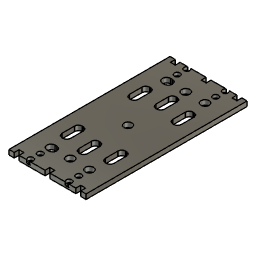
FS80+UL Pivot Base v20 (Autodesk Fusion 360 design; units mm, degrees)
Autodesk Fusion 360 part; units mm, degrees
note: some values were not read from the file. Set by a fixed rule: which sketch regions a step uses.
sketch "Schizzo5" plane through (0, 0, 0) normal (0, 0, 1) x (1, 0, 0)
  line L0 (214.6877, 113.6857) -> (294.6877, 113.6857)
  line L1 (294.6877, 113.6857) -> (294.6877, -53.5143)
  line L2 (294.6877, -53.5143) -> (214.6877, -53.5143)
  line L3 (214.6877, -53.5143) -> (214.6877, 113.6857)
  line L4 (254.6877, 113.6857) -> (254.6877, -53.5143) construction
  line L5 (214.6877, 30.0857) -> (294.6877, 30.0857) construction
  line L6 (274.6877, -51.0143) -> (234.6877, -51.0143) construction
  line L7 (234.6877, -51.0143) -> (234.6877, -41.0143) construction
  line L8 (234.6877, -41.0143) -> (274.6877, -41.0143) construction
  line L9 (274.6877, -41.0143) -> (274.6877, -51.0143) construction
  line L10 (274.6877, -51.0143) -> (234.6877, -41.0143) construction
  line L11 (234.6877, -51.0143) -> (274.6877, -41.0143) construction
  line L12 (225.2377, -53.5143) -> (220.1377, -53.5143)
  line L13 (220.1377, -53.5143) -> (220.1377, -48.5143)
  line L14 (220.1377, -48.5143) -> (225.2377, -48.5143)
  line L15 (225.2377, -48.5143) -> (225.2377, -53.5143)
  line L16 (225.2377, -53.5143) -> (220.1377, -48.5143) construction
  line L17 (220.1377, -53.5143) -> (225.2377, -48.5143) construction
  line L18 (289.2377, -48.5143) -> (284.1377, -48.5143)
  line L19 (289.2377, -53.5143) -> (289.2377, -48.5143)
  line L20 (284.1377, -48.5143) -> (284.1377, -53.5143)
  line L21 (284.1377, -53.5143) -> (289.2377, -53.5143)
  circle A0 centre (234.6877, -41.0143) radius 1.6
  circle A1 centre (234.6877, -41.0143) radius 2.95
  line L22 (234.6877, -46.0143) -> (274.6877, -46.0143) construction
  circle A2 centre (234.6877, -51.0143) radius 1.6
  circle A3 centre (234.6877, -51.0143) radius 2.95
  circle A4 centre (274.6877, -41.0143) radius 2.95
  circle A5 centre (274.6877, -41.0143) radius 1.6
  circle A6 centre (274.6877, -51.0143) radius 1.6
  circle A7 centre (274.6877, -51.0143) radius 2.95
  circle A8 centre (234.6877, 111.1857) radius 2.95
  circle A9 centre (234.6877, 111.1857) radius 1.6
  circle A10 centre (234.6877, 101.1857) radius 2.95
  circle A11 centre (234.6877, 101.1857) radius 1.6
  circle A12 centre (274.6877, 101.1857) radius 2.95
  circle A13 centre (274.6877, 101.1857) radius 1.6
  circle A14 centre (274.6877, 111.1857) radius 2.95
  circle A15 centre (274.6877, 111.1857) radius 1.6
  line L23 (289.2377, 108.6857) -> (284.1377, 108.6857)
  line L24 (284.1377, 108.6857) -> (284.1377, 113.6857)
  line L25 (289.2377, 113.6857) -> (289.2377, 108.6857)
  line L26 (225.2377, 108.6857) -> (225.2377, 113.6857)
  line L27 (220.1377, 108.6857) -> (225.2377, 108.6857)
  line L28 (220.1377, 113.6857) -> (220.1377, 108.6857)
  line L29 (257.2377, -53.5143) -> (252.1377, -53.5143)
  line L30 (252.1377, -53.5143) -> (252.1377, -48.5143)
  line L31 (252.1377, -48.5143) -> (257.2377, -48.5143)
  line L32 (257.2377, -48.5143) -> (257.2377, -53.5143)
  line L33 (257.2377, -53.5143) -> (252.1377, -48.5143) construction
  line L34 (252.1377, -53.5143) -> (257.2377, -48.5143) construction
  line L35 (252.1377, 108.6857) -> (257.2377, 108.6857)
  line L36 (252.1377, 113.6857) -> (252.1377, 108.6857)
  line L37 (257.2377, 108.6857) -> (257.2377, 113.6857)
  point P0 (254.6877, -46.0143)
  point P1 (222.6877, -51.0143)
  point P2 (286.6877, -51.0143)
  point P3 (222.6877, -51.0143)
  point P4 (254.6877, -51.0143)
  dimension "d398" = 80
  dimension "d399" = 167.2
  dimension "d400" = 40
  dimension "d401" = 10
  dimension "d402" = 2.5
  dimension "d403" = 64
  dimension "d404" = 5.1
  dimension "d405" = 5
  dimension "d406" = 3.2
  dimension "d407" = 5.9
  dimension "d410" = 5.1
  dimension "d411" = 5
  constraint horizontal L0
  constraint vertical L1
  constraint horizontal L2
  constraint vertical L3
  constraint midpoint L0 L4.start
  constraint midpoint L2 L4.end
  constraint midpoint L3 L5.start
  constraint midpoint L1 L5.end
  constraint horizontal L6
  constraint perpendicular L6 L7
  constraint parallel L6 L8
  constraint parallel L7 L9
  constraint coincident L10 P0
  constraint coincident L11 P0
  constraint coincident L4 P0
  constraint symmetric L4 P3 P2
  constraint coincident L6 P3
  constraint horizontal L12
  constraint perpendicular L12 L13
  constraint parallel L12 L14
  constraint parallel L13 L15
  constraint coincident L16 P3
  constraint coincident L17 P3
  constraint coincident P3 P1
  constraint symmetric L4 L12.start L20.end
  constraint symmetric L4 L12.end L19.start
  constraint symmetric L4 L13.end L18.start
  constraint symmetric L4 L14.end L18.end
  constraint coincident L7.end L8.start
  constraint concentric A0 A1
  constraint midpoint L7 L22.start
  constraint midpoint L9 L22.end
  constraint symmetric A0 L22 A2
  constraint symmetric A1 L22 A3
  constraint symmetric L4 A0 A5
  constraint symmetric L4 A1 A4
  constraint symmetric L4 A2 A6
  constraint symmetric L4 A3 A7
  constraint symmetric L5 L12.start L26.end
  constraint symmetric L5 L12.end L28.start
  constraint symmetric L5 L13.end L27.start
  constraint symmetric L5 L14.end L26.start
  constraint symmetric L5 L18.start L23.start
  constraint symmetric L5 L18.end L23.end
  constraint symmetric L5 L19.start L25.start
  constraint symmetric L5 L20.end L24.end
  constraint symmetric L5 A0 A11
  constraint symmetric L5 A1 A10
  constraint symmetric L5 A2 A9
  constraint symmetric L5 A3 A8
  constraint symmetric L5 A4 A12
  constraint symmetric L5 A5 A13
  constraint symmetric L5 A6 A15
  constraint symmetric L5 A7 A14
  constraint horizontal L29
  constraint perpendicular L29 L30
  constraint parallel L29 L31
  constraint parallel L30 L32
  constraint coincident L33 P4
  constraint coincident L34 P4
  constraint midpoint L6 P4
  constraint symmetric L5 L29.start L37.end
  constraint symmetric L5 L29.end L36.start
  constraint symmetric L5 L30.end L35.start
  constraint symmetric L5 L31.end L35.end
  measures "d398" distance of L0.start L0.end
  measures "d399" distance of L0.start L2.end
  measures "d400" distance of L7.end L8.end
  measures "d401" distance of L6.end L7.end
  measures "d402" distance of L2 L6
  measures "d403" distance of P3 P2
  measures "d404" distance of L13.end L14.end
  measures "d405" distance of L12.end L13.end
  measures "d406" diameter of A0
  measures "d407" diameter of A1
  measures "d410" distance of L30.end L31.end
  measures "d411" distance of L29.end L30.end
extrude "Estrusione32" add sketch "Schizzo5" along normal blind 5 contours L0 L1 L2 L3 L13 L14 L15 L18 L19 L20 A3 A7 A8 A14 L23 L24 L25 L26 L27 L28 L30 L31 L32 L35 L36 L37 | L0 L26 L27 L28 | L2 L12 L13 L14 L15 | L0 A8 | L2 A3 | L0 L35 L36 L37 | L2 L29 L30 L31 L32 | L0 A14 | L2 A7 | L0 L23 L24 L25 | L2 L18 L19 L20 L21 | A0 | A1 | A2 | A4 | A5 | A6 | A9 | A10 | A11 | A12 | A13 | A15 picked at (234.7276, 113.3842) picked at (234.7276, -53.2128) picked at (274.7276, 113.3842) picked at (274.6479, -53.2128)
sketch "Schizzo20" plane through (0, 0, 5) normal (0, 0, 1) x (-1, 0, 0)
  line L0 (-214.6877, 53.5143) -> (-294.6877, 53.5143)
  line L1 (-294.6877, 53.5143) -> (-294.6877, -113.6857)
  line L2 (-294.6877, -113.6857) -> (-214.6877, -113.6857)
  line L3 (-214.6877, -113.6857) -> (-214.6877, 53.5143)
  line L4 (-214.6877, -113.6857) -> (-294.6877, -113.6857) construction
  line L5 (-294.6877, -113.6857) -> (-294.6877, 53.5143) construction
  line L6 (-294.6877, 53.5143) -> (-214.6877, 53.5143) construction
  line L7 (-214.6877, 53.5143) -> (-214.6877, -113.6857) construction
  line L8 (-254.6877, -113.6857) -> (-254.6877, 53.5143) construction
  line L9 (-214.6877, -30.0857) -> (-294.6877, -30.0857) construction
  circle A0 centre (-254.6877, -30.0857) radius 4.1
  line L10 (-259.1877, -59.5857) -> (-250.1877, -59.5857)
  line L11 (-250.1877, -59.5857) -> (-250.1877, -80.5857)
  line L12 (-250.1877, -80.5857) -> (-259.1877, -80.5857)
  line L13 (-259.1877, -80.5857) -> (-259.1877, -59.5857)
  line L14 (-259.1877, -59.5857) -> (-250.1877, -80.5857) construction
  line L15 (-250.1877, -59.5857) -> (-259.1877, -80.5857) construction
  line L16 (-250.1877, -0.5857) -> (-250.1877, 20.4143)
  line L17 (-259.1877, 20.4143) -> (-259.1877, -0.5857)
  line L18 (-259.1877, -0.5857) -> (-250.1877, -0.5857)
  line L19 (-250.1877, 20.4143) -> (-259.1877, 20.4143)
  circle A1 centre (-254.6877, -90.0857) radius 4.25
  circle A2 centre (-254.6877, 29.9143) radius 4.25
  point P0 (-254.6877, -70.0857)
  point P1 (-254.6877, 9.9143)
  point P2 (-254.6877, -70.0857)
  dimension "d412" = 8.2
  dimension "d413" = 80
  dimension "d414" = 9
  dimension "d415" = 21
  dimension "d435" = 8.5
  dimension "d436" = 120
  constraint horizontal L4
  constraint vertical L5
  constraint horizontal L6
  constraint vertical L7
  constraint coincident L2.end L3.start
  constraint coincident L0.end L1.start
  constraint midpoint L4 L8.start
  constraint midpoint L6 L8.end
  constraint midpoint L7 L9.start
  constraint midpoint L5 L9.end
  constraint midpoint L9 A0.centre
  constraint coincident L8 P2
  constraint symmetric L9 P2 P1
  constraint horizontal L10
  constraint perpendicular L10 L11
  constraint parallel L10 L12
  constraint parallel L11 L13
  constraint coincident L14 P2
  constraint coincident L15 P2
  constraint coincident P2 P0
  constraint symmetric L9 L10.start L17.end
  constraint symmetric L9 L10.end L16.start
  constraint symmetric L9 L11.end L16.end
  constraint symmetric L9 L12.end L17.start
  constraint coincident L8 A1.centre
  constraint symmetric L9 A1 A2
  measures "d412" diameter of A0
  measures "d413" distance of P2 P1
  measures "d414" distance of L11.end L12.end
  measures "d415" distance of L10.end L11.end
  measures "d435" diameter of A1
  measures "d436" distance of A1.centre A2.centre
extrude "Estrusione33" cut sketch "Schizzo20" against normal blind 5 contours A0 | L10 L11 L12 L13 | L16 L17 L18 L19 | A1 | A2
fillet "Raccordo7" radius 4 4 edges at (250.1877, 0.5857, 2.5) (250.1877, -20.4143, 2.5) (259.1877, -20.4143, 2.5) (259.1877, 0.5857, 2.5)
fillet "Raccordo7" radius 4 4 edges at (250.1877, 59.5857, 2.5) (250.1877, 80.5857, 2.5) (259.1877, 80.5857, 2.5) (259.1877, 59.5857, 2.5)
sketch "Schizzo21" plane through (0, 0, 5) normal (0, 0, 1) x (-1, 0, 0)
  line L0 (-250.1877, -63.5857) -> (-250.1877, -76.5857)
  line L1 (-254.1877, -80.5857) -> (-255.1877, -80.5857)
  line L2 (-259.1877, -76.5857) -> (-259.1877, -63.5857)
  line L3 (-255.1877, -59.5857) -> (-254.1877, -59.5857)
  circle A0 centre (-254.6877, -30.0857) radius 4.1
  line L4 (-259.1877, 3.4143) -> (-259.1877, 16.4143)
  line L5 (-255.1877, 20.4143) -> (-254.1877, 20.4143)
  line L6 (-250.1877, 16.4143) -> (-250.1877, 3.4143)
  line L7 (-254.1877, -0.5857) -> (-255.1877, -0.5857)
  line L8 (-214.6877, 53.5143) -> (-294.6877, 53.5143)
  line L9 (-294.6877, 53.5143) -> (-294.6877, -113.6857)
  line L10 (-294.6877, -113.6857) -> (-214.6877, -113.6857)
  line L11 (-214.6877, -113.6857) -> (-214.6877, 53.5143)
  line L12 (-214.6877, -113.6857) -> (-294.6877, -113.6857) construction
  line L13 (-294.6877, -113.6857) -> (-294.6877, 53.5143) construction
  line L14 (-294.6877, 53.5143) -> (-214.6877, 53.5143) construction
  line L15 (-214.6877, 53.5143) -> (-214.6877, -113.6857) construction
  line L16 (-254.6877, -113.6857) -> (-254.6877, 53.5143) construction
  line L17 (-214.6877, -30.0857) -> (-294.6877, -30.0857) construction
  line L18 (-236.6877, -54.5857) -> (-227.6877, -54.5857)
  line L19 (-227.6877, -54.5857) -> (-227.6877, -75.5857)
  line L20 (-227.6877, -75.5857) -> (-236.6877, -75.5857)
  line L21 (-236.6877, -75.5857) -> (-236.6877, -54.5857)
  line L22 (-236.6877, -54.5857) -> (-227.6877, -75.5857) construction
  line L23 (-227.6877, -54.5857) -> (-236.6877, -75.5857) construction
  line L24 (-236.6877, 15.4143) -> (-236.6877, -5.5857)
  line L25 (-227.6877, 15.4143) -> (-236.6877, 15.4143)
  line L26 (-227.6877, -5.5857) -> (-227.6877, 15.4143)
  line L27 (-236.6877, -5.5857) -> (-227.6877, -5.5857)
  line L28 (-272.6877, -75.5857) -> (-272.6877, -54.5857)
  line L29 (-272.6877, -54.5857) -> (-281.6877, -54.5857)
  line L30 (-281.6877, -54.5857) -> (-281.6877, -75.5857)
  line L31 (-281.6877, -75.5857) -> (-272.6877, -75.5857)
  line L32 (-281.6877, 15.4143) -> (-272.6877, 15.4143)
  line L33 (-272.6877, 15.4143) -> (-272.6877, -5.5857)
  line L34 (-272.6877, -5.5857) -> (-281.6877, -5.5857)
  line L35 (-281.6877, -5.5857) -> (-281.6877, 15.4143)
  circle A1 centre (-254.6877, 29.9143) radius 4.25
  circle A2 centre (-254.6877, -90.0857) radius 4.25
  arc A3 (-255.1877, 20.4143) -> (-259.1877, 16.4143) centre (-255.1877, 16.4143) ccw
  arc A4 (-250.1877, 16.4143) -> (-254.1877, 20.4143) centre (-254.1877, 16.4143) ccw
  arc A5 (-254.1877, -0.5857) -> (-250.1877, 3.4143) centre (-254.1877, 3.4143) ccw
  arc A6 (-259.1877, 3.4143) -> (-255.1877, -0.5857) centre (-255.1877, 3.4143) ccw
  arc A7 (-254.1877, -80.5857) -> (-250.1877, -76.5857) centre (-254.1877, -76.5857) ccw
  arc A8 (-259.1877, -76.5857) -> (-255.1877, -80.5857) centre (-255.1877, -76.5857) ccw
  arc A9 (-255.1877, -59.5857) -> (-259.1877, -63.5857) centre (-255.1877, -63.5857) ccw
  arc A10 (-250.1877, -63.5857) -> (-254.1877, -59.5857) centre (-254.1877, -63.5857) ccw
  point P0 (-232.1877, -65.0857)
  point P1 (-232.1877, 4.9143)
  point P2 (-232.1877, -65.0857)
  point P3 (-277.1877, -65.0857)
  dimension "d418" = 70
  dimension "d419" = 9
  dimension "d420" = 21
  dimension "d421" = 45
  constraint horizontal L12
  constraint vertical L13
  constraint horizontal L14
  constraint vertical L15
  constraint coincident L10.end L11.start
  constraint coincident L8.end L9.start
  constraint midpoint L12 L16.start
  constraint midpoint L14 L16.end
  constraint midpoint L15 L17.start
  constraint midpoint L13 L17.end
  constraint symmetric L17 P2 P1
  constraint horizontal L18
  constraint perpendicular L18 L19
  constraint parallel L18 L20
  constraint parallel L19 L21
  constraint coincident L22 P2
  constraint coincident L23 P2
  constraint coincident P2 P0
  constraint symmetric L17 L18.start L24.end
  constraint symmetric L17 L18.end L26.start
  constraint symmetric L17 L19.end L25.start
  constraint symmetric L17 L20.end L24.start
  constraint symmetric L16 P2 P3
  constraint symmetric L16 L18.start L28.end
  constraint symmetric L16 L18.end L29.end
  constraint symmetric L16 L19.end L30.end
  constraint symmetric L16 L20.end L28.start
  constraint symmetric L16 L24.start L32.end
  constraint symmetric L16 L24.end L33.end
  constraint symmetric L16 L25.start L32.start
  constraint symmetric L16 L26.start L34.end
  measures "d418" distance of P2 P1
  measures "d419" distance of L19.end L20.end
  measures "d420" distance of L18.end L19.end
  measures "d421" distance of P2 P3
extrude "Estrusione34" cut sketch "Schizzo21" against normal blind 5 contours L18 L19 L20 L21 | L24 L25 L26 L27 | L28 L29 L30 L31 | L32 L33 L34 L35
fillet "Raccordo9" radius 4 4 edges at (227.6877, 5.5857, 2.5) (236.6877, 5.5857, 2.5) (236.6877, -15.4143, 2.5) (227.6877, -15.4143, 2.5)
fillet "Raccordo9" radius 4 4 edges at (227.6877, 75.5857, 2.5) (236.6877, 75.5857, 2.5) (236.6877, 54.5857, 2.5) (227.6877, 54.5857, 2.5)
fillet "Raccordo9" radius 4 4 edges at (272.6877, 5.5857, 2.5) (281.6877, 5.5857, 2.5) (281.6877, -15.4143, 2.5) (272.6877, -15.4143, 2.5)
fillet "Raccordo9" radius 4 4 edges at (272.6877, 75.5857, 2.5) (272.6877, 54.5857, 2.5) (281.6877, 54.5857, 2.5) (281.6877, 75.5857, 2.5)
sketch "Schizzo22" plane through (0, 0, 5) normal (0, 0, 1) x (-1, 0, 0)
  line L0 (-272.6877, -58.5857) -> (-272.6877, -71.5857)
  line L1 (-276.6877, -75.5857) -> (-277.6877, -75.5857)
  line L2 (-281.6877, -71.5857) -> (-281.6877, -58.5857)
  line L3 (-277.6877, -54.5857) -> (-276.6877, -54.5857)
  line L4 (-227.6877, 11.4143) -> (-227.6877, -1.5857)
  line L5 (-231.6877, -5.5857) -> (-232.6877, -5.5857)
  line L6 (-236.6877, -1.5857) -> (-236.6877, 11.4143)
  line L7 (-232.6877, 15.4143) -> (-231.6877, 15.4143)
  line L8 (-227.6877, -58.5857) -> (-227.6877, -71.5857)
  line L9 (-231.6877, -75.5857) -> (-232.6877, -75.5857)
  line L10 (-236.6877, -71.5857) -> (-236.6877, -58.5857)
  line L11 (-232.6877, -54.5857) -> (-231.6877, -54.5857)
  line L12 (-272.6877, 11.4143) -> (-272.6877, -1.5857)
  line L13 (-276.6877, -5.5857) -> (-277.6877, -5.5857)
  line L14 (-281.6877, -1.5857) -> (-281.6877, 11.4143)
  line L15 (-277.6877, 15.4143) -> (-276.6877, 15.4143)
  line L16 (-250.1877, -63.5857) -> (-250.1877, -76.5857)
  line L17 (-254.1877, -80.5857) -> (-255.1877, -80.5857)
  line L18 (-259.1877, -76.5857) -> (-259.1877, -63.5857)
  line L19 (-255.1877, -59.5857) -> (-254.1877, -59.5857)
  circle A0 centre (-254.6877, -30.0857) radius 4.1
  line L20 (-259.1877, 3.4143) -> (-259.1877, 16.4143)
  line L21 (-255.1877, 20.4143) -> (-254.1877, 20.4143)
  line L22 (-250.1877, 16.4143) -> (-250.1877, 3.4143)
  line L23 (-254.1877, -0.5857) -> (-255.1877, -0.5857)
  line L24 (-214.6877, 53.5143) -> (-294.6877, 53.5143)
  line L25 (-294.6877, 53.5143) -> (-294.6877, -113.6857)
  line L26 (-294.6877, -113.6857) -> (-214.6877, -113.6857)
  line L27 (-214.6877, -113.6857) -> (-214.6877, 53.5143)
  line L28 (-214.6877, -113.6857) -> (-294.6877, -113.6857) construction
  line L29 (-294.6877, -113.6857) -> (-294.6877, 53.5143) construction
  line L30 (-294.6877, 53.5143) -> (-214.6877, 53.5143) construction
  line L31 (-214.6877, 53.5143) -> (-214.6877, -113.6857) construction
  line L32 (-274.6877, -113.6857) -> (-274.6877, 53.5143) construction
  circle A1 centre (-234.6877, -90.0857) radius 4.25
  line L33 (-254.6877, -113.6857) -> (-254.6877, 53.5143) construction
  line L34 (-214.6877, -30.0857) -> (-294.6877, -30.0857) construction
  circle A2 centre (-274.6877, -90.0857) radius 4.25
  circle A3 centre (-274.6877, 29.9143) radius 4.25
  circle A4 centre (-234.6877, 29.9143) radius 4.25
  line L35 (-236.5877, -113.6857) -> (-236.5877, 53.5143) construction
  circle A5 centre (-236.5877, -90.0857) radius 4.25
  line L36 (-234.6877, -94.3357) -> (-234.6877, -85.8357) construction
  line L37 (-234.6877, -94.3357) -> (-236.5877, -94.3357)
  line L38 (-234.6877, -85.8357) -> (-236.5877, -85.8357)
  circle A6 centre (-236.5877, 29.9143) radius 4.25
  line L39 (-234.6877, 34.1643) -> (-236.5877, 34.1643)
  line L40 (-234.6877, 25.6643) -> (-236.5877, 25.6643)
  circle A7 centre (-254.6877, 29.9143) radius 4.25
  circle A8 centre (-254.6877, -90.0857) radius 4.25
  arc A9 (-276.6877, -75.5857) -> (-272.6877, -71.5857) centre (-276.6877, -71.5857) ccw
  arc A10 (-281.6877, -71.5857) -> (-277.6877, -75.5857) centre (-277.6877, -71.5857) ccw
  arc A11 (-277.6877, -54.5857) -> (-281.6877, -58.5857) centre (-277.6877, -58.5857) ccw
  arc A12 (-272.6877, -58.5857) -> (-276.6877, -54.5857) centre (-276.6877, -58.5857) ccw
  arc A13 (-231.6877, -5.5857) -> (-227.6877, -1.5857) centre (-231.6877, -1.5857) ccw
  arc A14 (-236.6877, -1.5857) -> (-232.6877, -5.5857) centre (-232.6877, -1.5857) ccw
  arc A15 (-232.6877, 15.4143) -> (-236.6877, 11.4143) centre (-232.6877, 11.4143) ccw
  arc A16 (-227.6877, 11.4143) -> (-231.6877, 15.4143) centre (-231.6877, 11.4143) ccw
  arc A17 (-231.6877, -75.5857) -> (-227.6877, -71.5857) centre (-231.6877, -71.5857) ccw
  arc A18 (-236.6877, -71.5857) -> (-232.6877, -75.5857) centre (-232.6877, -71.5857) ccw
  arc A19 (-232.6877, -54.5857) -> (-236.6877, -58.5857) centre (-232.6877, -58.5857) ccw
  arc A20 (-227.6877, -58.5857) -> (-231.6877, -54.5857) centre (-231.6877, -58.5857) ccw
  arc A21 (-276.6877, -5.5857) -> (-272.6877, -1.5857) centre (-276.6877, -1.5857) ccw
  arc A22 (-281.6877, -1.5857) -> (-277.6877, -5.5857) centre (-277.6877, -1.5857) ccw
  arc A23 (-277.6877, 15.4143) -> (-281.6877, 11.4143) centre (-277.6877, 11.4143) ccw
  arc A24 (-272.6877, 11.4143) -> (-276.6877, 15.4143) centre (-276.6877, 11.4143) ccw
  arc A25 (-255.1877, 20.4143) -> (-259.1877, 16.4143) centre (-255.1877, 16.4143) ccw
  arc A26 (-250.1877, 16.4143) -> (-254.1877, 20.4143) centre (-254.1877, 16.4143) ccw
  arc A27 (-254.1877, -0.5857) -> (-250.1877, 3.4143) centre (-254.1877, 3.4143) ccw
  arc A28 (-259.1877, 3.4143) -> (-255.1877, -0.5857) centre (-255.1877, 3.4143) ccw
  arc A29 (-254.1877, -80.5857) -> (-250.1877, -76.5857) centre (-254.1877, -76.5857) ccw
  arc A30 (-259.1877, -76.5857) -> (-255.1877, -80.5857) centre (-255.1877, -76.5857) ccw
  arc A31 (-255.1877, -59.5857) -> (-259.1877, -63.5857) centre (-255.1877, -63.5857) ccw
  arc A32 (-250.1877, -63.5857) -> (-254.1877, -59.5857) centre (-254.1877, -63.5857) ccw
  point P0 (-234.6877, 29.9143)
  dimension "d426" = 8.5
  dimension "d427" = 40
  dimension "d429" = 38.1
  dimension "d430" = 8.5
  dimension "d437" = 120
  dimension "d441" = 23.6
  constraint horizontal L28
  constraint vertical L29
  constraint horizontal L30
  constraint vertical L31
  constraint coincident L26.end L27.start
  constraint coincident L24.end L25.start
  constraint coincident L28 L32.start
  constraint coincident L30 L32.end
  constraint perpendicular L30 L32
  constraint midpoint L28 L33.start
  constraint midpoint L30 L33.end
  constraint midpoint L31 L34.start
  constraint midpoint L29 L34.end
  constraint symmetric A1 L33 A2
  constraint symmetric A1.centre L34 P0
  constraint symmetric L34 A2 A3
  constraint symmetric A1 L34 A4
  constraint coincident L32 A2.centre
  constraint coincident L28 L35.start
  constraint coincident L30 L35.end
  constraint perpendicular L30 L35
  constraint coincident L35 A5.centre
  constraint coincident A1 L36.start
  constraint coincident A1 L36.end
  constraint vertical L36
  constraint coincident A5 L37.end
  constraint coincident L35 L37.end
  constraint tangent A5 L37
  constraint coincident A5 L38.end
  constraint coincident L35 L38.end
  constraint tangent A5 L38
  constraint symmetric L34 A5 A6
  constraint symmetric L34 L36.start L39.start
  constraint symmetric L34 L36.end L40.start
  constraint symmetric L34 L37.end L39.end
  constraint symmetric L34 L38.end L40.end
  measures "d426" diameter of A1
  measures "d427" distance of A1.centre A2.centre
  measures "d429" distance of L32.start L35
  measures "d430" diameter of A5
  measures "d437" distance of A2.centre A3.centre
  measures "d441" distance of L30 A3.centre
extrude "Estrusione37" cut sketch "Schizzo22" against normal blind 5 contours A1 A5 | A1 A5 L38 | A1 A5 L37 | A1 A5 | A1 A5 | A2 | A3 | A4 A6 | A4 A6 L39 | A4 A6 L40 | A4 A6 | A4 A6
extrude "Estrusione38" cut sketch "Schizzo5" along normal blind 5 contours L0 L26 L27 L28 | L2 L12 L13 L14 L15 | L0 L35 L36 L37 | L2 L29 L30 L31 L32 | L0 L23 L24 L25 | L2 L18 L19 L20 L21 | A0 | A2 | A5 | A6 | A9 | A11 | A13 | A15
extrude "Estrusione35" cut sketch "Schizzo5" against normal blind 3.2 from surface at 5 contours L0 A8 | L2 A3 | L0 A14 | L2 A7 | A1 | A4 | A10 | A12 picked at (234.7276, 113.3842) picked at (234.7276, -53.2128) picked at (274.7276, 113.3842) picked at (274.6479, -53.2128)
named bodies: "Final"
